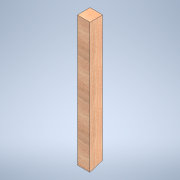
# Autodesk Inventor part: 4x4x36-post
Saved by Autodesk Inventor 2020.2 (Build 242310000, 310)
## iProperties
Created: 2020-03-27
Part Number: 4x4x36-post
Material: Wood (Birch)
Document SubType Name: Modeling
Designer: robst
Density: 0.55 g/cm^3
Appearance: Birch - Natural Polished
Author: robst
Autodesk Inventor part; units mm, degrees
ref_plane "YZ Plane" through (0, 0, 0) normal (1, 0, 0) x (0, 1, 0)
ref_plane "XZ Plane" through (0, 0, 0) normal (0, 1, 0) x (-1, 0, 0)
ref_plane "XY Plane" through (0, 0, 0) normal (0, 0, 1) x (1, 0, 0)
sketch "Sketch1" plane through (0, 0, 0) normal (1, 0, 0) x (0, 1, 0)
  line L0 (0, 0) -> (29.6333, -88.9)
  line L1 (29.6333, -88.9) -> (914.4, -88.9)
  line L2 (914.4, -88.9) -> (914.4, 0)
  line L3 (914.4, 0) -> (0, 0)
  line L4 (0, 0) -> (0, -88.9) construction
  dimension "width" = 88.9
  dimension "roofAngle" = 18.435
  dimension "height" = 914.4
  constraints: 10 end point, 2 perpendicular, 1 horizontal, 1 vertical
  measures "width" distance between parallel lines of L1 L3
  measures "roofAngle" angle of L0 L4
  measures "height" distance of L2.end L0.start
extrude "Extrusion1" add sketch "Sketch1" along normal mid plane 88.9
equation "\"d3\" = width"
body "Solid1"
